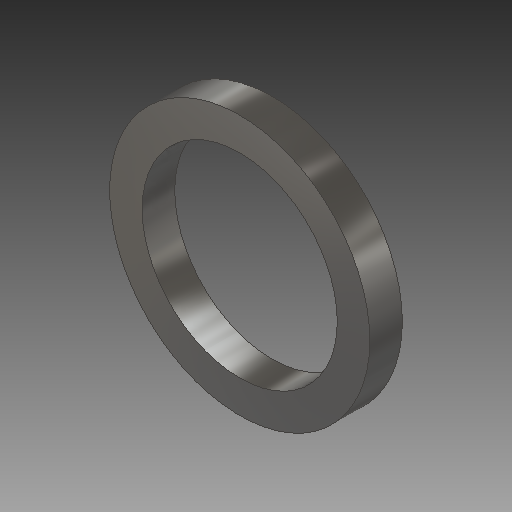
# Autodesk Inventor part: シムリング0608,1t
Saved by Autodesk Inventor 2019 (Build 230136000, 136)
## iProperties
Created: 2018-09-06
Part Number: シムリング0608,1t
Material: 鋼、高強度、低合金
Document SubType Name: Modeling
Designer: 雪村
Density: 7.85 g/cm^3
Appearance: 鋼 - つや出し
Mass: 0.172631 g
Surface Area: 0.879646 cm^2
Volume: 0.0219911 cm^3
Author: 雪村
Autodesk Inventor part; units mm, degrees
ref_plane "YZ Plane" through (0, 0, 0) normal (1, 0, 0) x (0, 1, 0)
ref_plane "XZ Plane" through (0, 0, 0) normal (0, 1, 0) x (-1, 0, 0)
ref_plane "XY Plane" through (0, 0, 0) normal (0, 0, 1) x (1, 0, 0)
sketch "スケッチ1" plane through (0, 0, 0) normal (0, 0, 1) x (1, 0, 0)
  circle A0 centre (0, 0) radius 3
  circle A1 centre (0, 0) radius 4
  dimension "d0" = 6
  dimension "d1" = 8
  constraints: 2 centre point, 2 coincident
  measures "d0" diameter of A0
  measures "d1" diameter of A1
extrude "押し出し1" add sketch "スケッチ1" along normal blind 1
